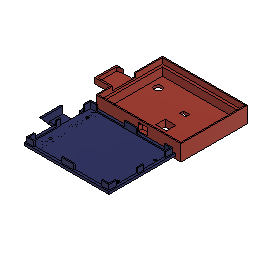
karpiu obudowa (Autodesk Fusion 360 design; units mm, degrees)
part number: Konfiguracja 1
Autodesk Fusion 360 part; units mm, degrees
note: some values were not read from the file. Chosen so that the rebuilt part matches the saved one: which bodies a step acts on; a direction; the layout of a text. Set by a fixed rule: which sketch regions a step uses.
sketch "Szkic1" plane through (0, 0, 0) normal (0, 0, 1) x (1, 0, 0)
  line L0 (65, 50) -> (-65, 50)
  line L1 (-65, 50) -> (-65, -50)
  line L2 (-65, -50) -> (65, -50)
  line L3 (65, -50) -> (65, 50)
  line L4 (-69, -54) -> (69, -54)
  line L5 (69, -54) -> (69, 54)
  line L6 (69, 54) -> (-69, 54)
  line L7 (-69, 54) -> (-69, -54)
  line L8 (-65, 28.5) -> (-91.3384, 28.5)
  line L9 (-91.3384, 28.5) -> (-91.3384, -1.5)
  line L10 (-91.3384, -1.5) -> (-65, -1.5)
  line L11 (-69, 31) -> (-95, 31)
  line L12 (-95, 31) -> (-95, -4)
  line L13 (-95, -4) -> (-69, -4)
  dimension "d100" = 35
  dimension "d101" = 30
  dimension "d102" = 2.5
  dimension "d103" = 100
  dimension "d104" = 130
  constraint horizontal L0
  constraint vertical L1
  constraint horizontal L2
  constraint vertical L3
  constraint horizontal L4
  constraint vertical L5
  constraint horizontal L6
  constraint vertical L7
  constraint coincident L1 L8.start
  constraint perpendicular L7 L8
  constraint perpendicular L8 L9
  constraint coincident L1 L10.end
  constraint perpendicular L1 L10
  constraint coincident L7 L11.start
  constraint perpendicular L7 L11
  constraint perpendicular L8 L12
  constraint coincident L7 L13.end
  constraint perpendicular L7 L13
  measures "d100" distance of L11.end L12.end
  measures "d101" distance of L8.end L9.end
  measures "d102" distance of L10 L13
  measures "d103" distance of L0.start L2.end
  measures "d104" distance of L1.end L2.end
extrude "Wyciągnięcie proste1" add sketch "Szkic1" along normal blind 25 contours L0 L1 L2 L3 L4 L5 L6 L7 L8 L10 | L7 L8 L9 L10 L11 L12 L13 makes body 1
sketch "Szkic2" plane through (0, 0, 25) normal (0, 0, 1) x (-1, 0, 0)
  line L0 (65, 1.5) -> (91.3384, 1.5)
  line L1 (91.3384, 1.5) -> (91.3384, -28.5)
  line L2 (91.3384, -28.5) -> (65, -28.5)
  line L3 (65, -28.5) -> (65, -50)
  line L4 (65, -50) -> (-65, -50)
  line L5 (-65, -50) -> (-65, 50)
  line L6 (-65, 50) -> (65, 50)
  line L7 (65, 50) -> (65, 1.5)
  line L8 (95, 4) -> (69, 4)
  line L9 (69, 4) -> (69, 54)
  line L10 (69, 54) -> (-69, 54)
  line L11 (-69, 54) -> (-69, -54)
  line L12 (-69, -54) -> (69, -54)
  line L13 (69, -54) -> (69, -31)
  line L14 (69, -31) -> (95, -31)
  line L15 (95, -31) -> (95, 4)
  line L16 (-17, -26) -> (0, -26)
  line L17 (0, -26) -> (0, -43)
  line L18 (0, -43) -> (-17, -43)
  line L19 (-17, -43) -> (-17, -26)
  constraint horizontal L16
  constraint vertical L17
  constraint horizontal L18
  constraint vertical L19
extrude "Wyciągnięcie proste2" add sketch "Szkic2" against normal blind 3 contours L0 L1 L2 L3 L4 L5 L6 L7 bodies 1
extrude "Wyciągnięcie proste3" add 1 faces at (0, -27.3333, 25) along direction (0, 0, 1) blind 1 on bodies 1 bodies 1
sketch "Szkic3" plane through (0, 0, 0) normal (0, 0, -1) x (1, 0, 0)
  line L0 (-65, 1.5) -> (-65, 50)
  line L1 (-65, 50) -> (65, 50)
  line L2 (65, 50) -> (65, -50)
  line L3 (65, -50) -> (-65, -50)
  line L4 (-65, -50) -> (-65, -28.5)
  line L5 (-91.3384, -28.5) -> (-91.3384, 1.5)
  line L6 (-95, -31) -> (-69, -31)
  line L7 (-69, -31) -> (-69, -54)
  line L8 (-69, -54) -> (69, -54)
  line L9 (69, -54) -> (69, 54)
  line L10 (69, 54) -> (-69, 54)
  line L11 (-69, 54) -> (-69, 4)
sketch "Szkic4" plane through (0, 0, 26) normal (0, 0, 1) x (-1, 0, 0)
  line L0 (0, -43) -> (-17, -43)
  line L1 (-17, -43) -> (-17, -26)
  line L2 (-17, -26) -> (0, -26)
  line L3 (0, -26) -> (0, -43)
  line L4 (95, 4) -> (69, 4)
  line L5 (69, 4) -> (69, 54)
  line L6 (69, 54) -> (-69, 54)
  line L7 (-69, 54) -> (-69, -54)
  line L8 (-69, -54) -> (69, -54)
  line L9 (69, -54) -> (69, -31)
  line L10 (69, -31) -> (95, -31)
  line L11 (95, -31) -> (95, 4)
  line L12 (69, -31) -> (69, 4)
  constraint coincident L9.end L10.start
  constraint coincident L4.end L5.start
extrude "Wyciągnięcie proste4" cut sketch "Szkic4" against normal blind 20 contours L4 L10 L11 L12 bodies 1
sketch "Szkic5" plane through (0, 0, 6) normal (0, 0, 1) x (-1, 0, 0)
  line L0 (91.3384, -28.5) -> (69, -28.5)
  line L1 (69, -28.5) -> (69, -31)
  line L2 (69, -31) -> (95, -31)
  line L3 (95, -31) -> (95, 4)
  line L4 (95, 4) -> (69, 4)
  line L5 (69, 4) -> (69, 1.5)
  line L6 (69, 1.5) -> (91.3384, 1.5)
  line L7 (91.3384, 1.5) -> (91.3384, -28.5)
  line L8 (69, -28.5) -> (69, 1.5)
  constraint coincident L0.end L1.start
  constraint coincident L5.end L6.start
extrude "Wyciągnięcie proste5" add sketch "Szkic5" along normal blind 3 separate body contours L0 L6 L7 L8 makes body 2
extrude "Wyciągnięcie proste6" add 1 faces at (-93.7795, 18.5, 6) along direction (0, 0, 1) blind 3 on bodies 1 bodies 1 2
sketch "Szkic6" plane through (-69, 0, 0) normal (-1, 0, 0) x (0, -1, 0)
  line L0 (4, 9) -> (4, 0)
  line L1 (4, 0) -> (54, 0)
  line L2 (54, 0) -> (54, 26)
  line L3 (54, 26) -> (-54, 26)
  line L4 (-54, 26) -> (-54, 0)
  line L5 (-54, 0) -> (-31, 0)
  line L6 (-31, 0) -> (-31, 9)
  line L7 (-31, 9) -> (-28.5, 9)
  line L8 (-28.5, 9) -> (-28.5, 22)
  line L9 (-28.5, 22) -> (1.5, 22)
  line L10 (1.5, 22) -> (1.5, 9)
  line L11 (1.5, 9) -> (4, 9)
  line L12 (-28.5, 9) -> (1.5, 9)
  constraint coincident L7.end L8.start
  constraint coincident L10.end L11.start
sketch "Szkic7" plane through (0, -4, 0) normal (0, -1, 0) x (1, 0, 0)
  line L0 (-95, 9) -> (-95, 0)
  line L1 (-95, 0) -> (-69, 0)
  line L2 (-69, 0) -> (-69, 9)
  line L3 (-69, 9) -> (-95, 9)
  line L4 (-90, 0) -> (-90, -11)
  line L5 (-90, -11) -> (-67, -11)
  line L6 (-67, -11) -> (-67, 0)
  line L7 (-90, 0) -> (-94, 0)
  line L8 (-94, 0) -> (-94, -15)
  line L9 (-94, -15) -> (-63, -15)
  line L10 (-63, -15) -> (-63, 0)
  line L11 (-63, 0) -> (-67, 0)
  constraint coincident L1 L4.start
  constraint perpendicular L1 L4
  constraint perpendicular L4 L5
  constraint perpendicular L5 L6
  constraint coincident L1 L7.end
  constraint perpendicular L1 L8
  constraint perpendicular L8 L9
  constraint perpendicular L9 L10
  constraint perpendicular L6 L11
extrude "Wyciągnięcie proste8" add sketch "Szkic7" against normal blind 35 contours L1 L4 L5 L6 L7 L8 L9 L10 L11 bodies 1
sketch "Szkic8" plane through (0, -4, 0) normal (0, -1, 0) x (1, 0, 0)
  line L0 (-95, 9) -> (-95, 0)
  line L1 (-95, 0) -> (-94, 0)
  line L2 (-94, 0) -> (-94, -15)
  line L3 (-94, -15) -> (-63, -15)
  line L4 (-63, -15) -> (-63, 0)
  line L5 (-63, 0) -> (-65, 0)
  line L6 (-65, 0) -> (-67, 0)
  line L7 (-67, 0) -> (-67, -11)
  line L8 (-67, -11) -> (-90, -11)
  line L9 (-90, -11) -> (-90, 0)
  line L10 (-90, 0) -> (-69, 0)
  line L11 (-69, 0) -> (-69, 9)
  line L12 (-69, 9) -> (-95, 9)
  line L13 (-63, 0) -> (-67, 0)
  line L14 (-90, 0) -> (-94, 0)
  line L15 (-94, 0) -> (-94, 9)
  constraint coincident L4.end L5.start
  constraint coincident L6.end L7.start
  constraint coincident L9.end L10.start
  constraint coincident L1.end L2.start
  constraint coincident L12 L15.end
  constraint perpendicular L12 L15
extrude "Wyciągnięcie proste9" cut sketch "Szkic8" against normal blind 13 contours L0 L1 L12 L15 | L2 L3 L4 L5 L6 L7 L8 L9 L13 L14 bodies 1
extrude "Wyciągnięcie proste10" cut 1 faces at (-94.3333, 9, 6) along direction (0, 1, 0) blind 23 on bodies 1 bodies 1
sketch "Szkic9" plane through (0, 9, 0) normal (0, -1, 0) x (1, 0, 0)
  line L0 (-91.3384, 0) -> (-94, 0)
  line L1 (-94, 0) -> (-94, -15)
  line L2 (-94, -15) -> (-63, -15)
  line L3 (-63, -15) -> (-63, 0)
  line L4 (-67, 0) -> (-67, -11)
  line L5 (-67, -11) -> (-90, -11)
  line L6 (-90, -11) -> (-90, 0)
  line L7 (-90, 0) -> (-91.3384, 0)
  line L8 (-67, 0) -> (-67, -0.1)
  line L9 (-67, -0.1) -> (-63, -0.1)
  line L10 (-63, 0) -> (-67, 0)
  constraint coincident L4.start L8.start
  constraint coincident L4 L8.end
  constraint coincident L3 L9.end
  constraint perpendicular L3 L9
extrude "Wyciągnięcie proste11" cut sketch "Szkic9" against normal blind 30 contours L3 L4 L8 L9 L10 bodies 1
sketch "Szkic10" plane through (0, 0, 22) normal (0, 0, -1) x (1, 0, 0)
  line L0 (-69, 1.5) -> (-69, -28.5)
  line L1 (-69, -28.5) -> (-65, -28.5)
  line L2 (-65, -28.5) -> (-65, -50)
  line L3 (-65, -50) -> (65, -50)
  line L4 (65, -50) -> (65, 50)
  line L5 (65, 50) -> (-65, 50)
  line L6 (-65, 50) -> (-65, 1.5)
  line L7 (-65, 1.5) -> (-69, 1.5)
  line L8 (17, -43) -> (0, -43)
  line L9 (0, -43) -> (0, -26)
  line L10 (0, -26) -> (17, -26)
  line L11 (17, -26) -> (17, -43)
  line L12 (-65, 1.5) -> (-65, -32)
  constraint coincident L6.end L7.start
  constraint coincident L2 L12.end
extrude "Wyciągnięcie proste12" add sketch "Szkic10" along normal blind 16 contours L0 L1 L7 L12 bodies 1
sketch "Szkic11" plane through (0, 0, 0) normal (0, 0, -1) x (1, 0, 0)
sketch "Szkic12" plane through (0, 0, 0) normal (0, 0, -1) x (1, 0, 0)
sketch "Szkic13" plane through (0, 0, -11) normal (0, 0, 1) x (-1, 0, 0)
  line L0 (90, -9) -> (67, -9)
  line L1 (67, -9) -> (67, -31)
  line L2 (67, -31) -> (90, -31)
  line L3 (90, -31) -> (90, -9)
  line L4 (90, -31) -> (67, -31)
  line L5 (67, -31) -> (67, -28)
  line L6 (67, -28) -> (90, -28)
  line L7 (90, -28) -> (90, -31)
  constraint horizontal L4
  constraint vertical L5
  constraint horizontal L6
  constraint vertical L7
  constraint coincident L1 L5.end
  constraint coincident L2.end L3.start
extrude "Wyciągnięcie proste13" add sketch "Szkic13" along normal blind 11 contours L1 L2 L3 L4 L5 L6 L7 bodies 1
sketch "Szkic14" plane through (-94, 0, 0) normal (-1, 0, 0) x (0, -1, 0)
  line L0 (-9, -15) -> (-9, 0)
  line L1 (-9, 0) -> (4, 0)
  line L2 (4, 0) -> (4, 9)
  line L3 (4, 9) -> (-31, 9)
  line L4 (-31, 9) -> (-31, -15)
  line L5 (-31, -15) -> (-9, -15)
  line L6 (-9, -15) -> (4, 0)
  constraint coincident L0.start L5.end
  constraint coincident L1.end L2.start
extrude "Wyciągnięcie proste14" add sketch "Szkic14" against normal blind 3 contours L0 L1 L6 bodies 1
extrude "Wyciągnięcie proste15" cut 1 faces at (-90, 15.3333, -3.6667) along direction (-1, 0, 0) blind 1 on bodies 1 bodies 1
extrude "Wyciągnięcie proste16" cut 1 faces at (-67, 15.3333, -7.3667) along direction (1, 0, 0) blind 1 on bodies 1 bodies 1
sketch "Szkic15" plane through (-63, 0, 0) normal (1, 0, 0) x (0, 1, 0)
  line L0 (31, -0.1) -> (9, -0.1)
  line L1 (9, -0.1) -> (9, -15)
  line L2 (9, -15) -> (31, -15)
  line L3 (31, -15) -> (31, -0.1)
  line L4 (9, -15) -> (2.043, 0.0231)
  line L5 (9, -0.1) -> (2.1, -0.1)
  constraint coincident L1.end L2.start
  constraint coincident L0.end L1.start
  constraint coincident L4 L5.end
  constraint perpendicular L1 L5
extrude "Wyciągnięcie proste17" add sketch "Szkic15" against normal blind 3 contours L1 L4 L5 bodies 1
sketch "Szkic16" plane through (-94, 0, 0) normal (-1, 0, 0) x (0, -1, 0)
  line L0 (4, 0) -> (4, 9)
  line L1 (4, 9) -> (-31, 9)
  line L2 (-31, 9) -> (-31, -15)
  line L3 (-31, -15) -> (-9, -15)
  line L4 (-9, -15) -> (4, 0)
  line L5 (4, 0) -> (-31, 0)
  line L6 (-31, 0) -> (-31, -0.1)
  line L7 (-31, -0.1) -> (4, -0.1)
  line L8 (4, -0.1) -> (4, 0)
  constraint horizontal L5
  constraint vertical L6
  constraint horizontal L7
  constraint vertical L8
  constraint coincident L2 L6.end
  constraint coincident L0.start L4.end
extrude "Wyciągnięcie proste18" cut sketch "Szkic16" against normal blind 51 contours L2 L4 L5 L6 L7 bodies 1 makes body 3 at (-74.3333, 23.6667, -15)
move_body "Przesuń1" bodies 3 to x (1, 0, 0) y (0, 1, 0) z (0, 0, 1) at (0, 0, -6)
sketch "Szkic17" plane through (0, 0, -6.1) normal (0, 0, 1) x (-1, 0, 0)
  line L0 (66, -28) -> (66, -2.1)
  line L1 (66, -2.1) -> (63, -2.1)
  line L2 (63, -2.1) -> (63, -31)
  line L3 (63, -31) -> (94, -31)
  line L4 (69, -31) -> (69, -54)
  line L5 (69, -54) -> (-69, -54)
  line L6 (-69, -54) -> (-69, 54)
  line L7 (-69, 54) -> (69, 54)
  line L8 (69, 54) -> (69, -2)
  line L9 (69, -2) -> (66, -2.1)
  line L10 (91, -28) -> (66, -28)
  line L11 (94, -31) -> (94, 3.9133)
  line L12 (94, 3.9133) -> (91, 3.9133)
  line L13 (91, 3.9133) -> (91, -28)
  constraint coincident L3 L4.start
  constraint perpendicular L3 L4
  constraint perpendicular L4 L5
  constraint perpendicular L5 L6
  constraint perpendicular L6 L7
  constraint perpendicular L7 L8
  constraint coincident L0.end L1.start
extrude "Wyciągnięcie proste19" add sketch "Szkic17" against normal blind 2 separate body contours L1 L2 L3 L4 L5 L6 L7 L8 L9 makes body 4
extrude "Wyciągnięcie proste20" add 1 faces at (-63, 11.7333, -6.7667) along direction (-1, 0, 0) blind 3 on bodies 4 bodies 3 4
sketch "Szkic18" plane through (0, 0, -6.1) normal (0, 0, 1) x (-1, 0, 0)
  line L0 (66, -2.1) -> (69, -2)
  line L1 (69, -2) -> (69, 54)
  line L2 (69, 54) -> (-69, 54)
  line L3 (-69, 54) -> (-69, -54)
  line L4 (-69, -54) -> (69, -54)
  line L5 (69, -54) -> (69, -31)
  line L6 (66, -28) -> (66, -2.1)
  line L7 (-65, 50) -> (65, 50)
  line L8 (65, 50) -> (65, -50)
  line L9 (65, -50) -> (-65, -50)
  line L10 (-65, -50) -> (-65, 50)
  line L11 (69, -31) -> (69, -28)
  line L12 (69, -28) -> (65, -28)
  line L13 (69, -2) -> (65, -2)
  line L14 (69, -31) -> (94, -31)
  line L15 (94, -31) -> (94, 3.9133)
  line L16 (94, 3.9133) -> (91, 3.9133)
  line L17 (91, 3.9133) -> (91, -28)
  line L18 (91, -28) -> (66, -28)
  constraint horizontal L7
  constraint vertical L8
  constraint horizontal L9
  constraint vertical L10
  constraint coincident L5.end L11.start
  constraint coincident L8 L12.end
  constraint perpendicular L8 L12
  constraint coincident L0.end L1.start
  constraint coincident L8 L13.end
  constraint perpendicular L8 L13
extrude "Wyciągnięcie proste21" add sketch "Szkic18" along normal blind 2 contours L1 L2 L3 L4 L5 L7 L8 L9 L10 L11 L12 L13 L18 bodies 3
sketch "Szkic19" plane through (0, 0, -4.1) normal (0, 0, 1) x (-1, 0, 0)
  line L0 (69, 54) -> (-69, 54)
  line L1 (-69, 54) -> (-69, -54)
  line L2 (-69, -54) -> (69, -54)
  line L3 (69, -54) -> (69, -28)
  line L4 (69, -28) -> (65, -28)
  line L5 (65, -28) -> (65, -50)
  line L6 (65, -50) -> (-65, -50)
  line L7 (-65, -50) -> (-65, 50)
  line L8 (-65, 50) -> (65, 50)
  line L9 (65, 50) -> (65, -2)
  line L10 (65, -2) -> (69, -2)
  line L11 (69, -2) -> (69, 54)
  line L12 (67, -52) -> (-67, -52)
  line L13 (-67, -52) -> (-67, 52)
  line L14 (-67, 52) -> (67, 52)
  line L15 (67, 52) -> (67, -52)
  constraint horizontal L12
  constraint vertical L13
  constraint horizontal L14
  constraint vertical L15
extrude "Wyciągnięcie proste22" add sketch "Szkic19" along normal blind 8 contours L4 L5 L6 L7 L8 L9 L10 L12 L13 L14 L15 bodies 3
sketch "Szkic20" plane through (0, 0, 3.9) normal (0, 0, 1) x (-1, 0, 0)
  line L0 (67, -28) -> (65, -28)
  line L1 (65, -28) -> (65, -50)
  line L2 (65, -50) -> (-65, -50)
  line L3 (-65, -50) -> (-65, 50)
  line L4 (-65, 50) -> (65, 50)
  line L5 (65, 50) -> (65, -2)
  line L6 (65, -2) -> (67, -2)
  line L7 (67, -2) -> (67, 52)
  line L8 (67, 52) -> (-67, 52)
  line L9 (-67, 52) -> (-67, -52)
  line L10 (-67, -52) -> (67, -52)
  line L11 (67, -52) -> (67, -28)
  line L12 (65, 40) -> (67, 40)
  line L13 (55, 50) -> (55, 52)
  line L14 (-55, 50) -> (-55, 52)
  line L15 (-65, 40) -> (-67, 40)
  line L16 (-65, -40) -> (-67, -40)
  line L17 (-55, -50) -> (-55, -52)
  line L18 (55, -50) -> (55, -52)
  line L19 (65, -40) -> (67, -40)
  line L20 (10, -52) -> (10, -50)
  line L21 (-10, -52) -> (-10, -50)
  line L22 (10, 50) -> (10, 52)
  line L23 (-10, 50) -> (-10, 52)
  line L24 (-65, 5) -> (-67, 5)
  line L25 (-65, -5) -> (-67, -5)
  line L26 (65, 5) -> (67, 5)
  constraint coincident L5 L12.start
  constraint coincident L7 L12.end
  constraint perpendicular L7 L12
  constraint coincident L4 L13.start
  constraint coincident L8 L13.end
  constraint perpendicular L8 L13
  constraint coincident L4 L14.start
  constraint coincident L8 L14.end
  constraint perpendicular L8 L14
  constraint coincident L3 L15.start
  constraint coincident L9 L15.end
  constraint perpendicular L9 L15
  constraint coincident L3 L16.start
  constraint coincident L9 L16.end
  constraint perpendicular L9 L16
  constraint coincident L2 L17.start
  constraint coincident L10 L17.end
  constraint perpendicular L10 L17
  constraint coincident L2 L18.start
  constraint coincident L10 L18.end
  constraint perpendicular L10 L18
  constraint coincident L1 L19.start
  constraint midpoint L11 L19.end
  constraint perpendicular L11 L19
  constraint coincident L10 L20.start
  constraint coincident L2 L20.end
  constraint perpendicular L2 L20
  constraint coincident L10 L21.start
  constraint coincident L2 L21.end
  constraint perpendicular L2 L21
  constraint coincident L4 L22.start
  constraint coincident L8 L22.end
  constraint perpendicular L8 L22
  constraint coincident L4 L23.start
  constraint coincident L8 L23.end
  constraint perpendicular L8 L23
  constraint coincident L3 L24.start
  constraint coincident L9 L24.end
  constraint perpendicular L9 L24
  constraint coincident L3 L25.start
  constraint coincident L9 L25.end
  constraint perpendicular L3 L25
  constraint coincident L5 L26.start
  constraint coincident L7 L26.end
  constraint perpendicular L7 L26
extrude "Wyciągnięcie proste23" cut sketch "Szkic20" against normal blind 8 contours L0 L1 L11 L19 | L2 L10 L18 L20 | L2 L10 L17 L21 | L3 L9 L16 L25 | L3 L9 L15 L24 | L4 L8 L14 L23 | L4 L8 L13 L22 | L5 L7 L12 L26 bodies 3
sketch "Szkic21" plane through (0, 0, 0) normal (0, 0, -1) x (1, 0, 0)
  line L0 (-91.3384, 1.5) -> (-65, 1.5)
  line L1 (-65, 1.5) -> (-65, 50)
  line L2 (-65, 50) -> (65, 50)
  line L3 (65, 50) -> (65, -50)
  line L4 (65, -50) -> (-65, -50)
  line L5 (-65, -50) -> (-65, -28.5)
  line L6 (-65, -28.5) -> (-91.3384, -28.5)
  line L7 (-91.3384, -28.5) -> (-91.3384, 1.5)
  line L8 (-69, 4) -> (-94, 4)
  line L9 (-94, 4) -> (-94, -31)
  line L10 (-94, -31) -> (-69, -31)
  line L11 (-69, -31) -> (-69, -54)
  line L12 (-69, -54) -> (69, -54)
  line L13 (69, -54) -> (69, 54)
  line L14 (69, 54) -> (-69, 54)
  line L15 (-69, 54) -> (-69, 4)
  line L16 (67.2, 52.2) -> (-67.2, 52.2)
  line L17 (-67.2, 52.2) -> (-67.2, -52.2)
  line L18 (-67.2, -52.2) -> (67.2, -52.2)
  line L19 (67.2, -52.2) -> (67.2, 52.2)
  constraint horizontal L16
  constraint vertical L17
  constraint horizontal L18
  constraint vertical L19
extrude "Wyciągnięcie proste24" cut sketch "Szkic21" against normal blind 9 contours L0 L1 L2 L3 L4 L5 L6 L16 L17 L18 L19 bodies 1
sketch "Szkic22" plane through (0, 0, 6) normal (0, 0, -1) x (1, 0, 0)
  line L0 (-67.2, -28.5) -> (-65, -28.5)
  line L1 (-65, -28.5) -> (-65, 1.5)
  line L2 (-65, 1.5) -> (-67.2, 1.5)
  line L3 (-67.2, 1.5) -> (-91.3384, 1.5)
  line L4 (-91.3384, 1.5) -> (-91.3384, -28.5)
  line L5 (-91.3384, -28.5) -> (-67.2, -28.5)
  line L6 (-67.2, 1.5) -> (-67.2, -28.5)
  constraint coincident L2.end L3.start
  constraint coincident L0.start L5.end
extrude "Wyciągnięcie proste25" cut sketch "Szkic22" against normal blind 3 contours L0 L1 L2 L6 bodies 1
extrude "Wyciągnięcie proste26" cut 1 faces at (0, 31.6667, 24.6667) along direction (-1, 0, 0) blind 0.2 on bodies 1 bodies 1
extrude "Wyciągnięcie proste27" cut 1 faces at (5.5333, 26, 24.6667) along direction (0, -1, 0) blind 0.2 on bodies 1 bodies 1
extrude "Wyciągnięcie proste28" cut 1 faces at (5.5333, 43, 23.3333) along direction (0, 1, 0) blind 0.2 on bodies 1 bodies 1
extrude "Wyciągnięcie proste29" cut 1 faces at (17, 31.6, 24.6667) along direction (1, 0, 0) blind 0.2 on bodies 1 bodies 1
move_body "Przesuń2" bodies 1 to x (1, 0, 0) y (0, -1, 0) z (0, 0, -1) at (0, 117, 26)
move_body "Przesuń3" bodies 3 to x (1, 0, 0) y (0, 1, 0) z (0, 0, 1) at (0, 0, 21)
sketch "Szkic23" plane through (0, 67, 0) normal (0, 1, 0) x (-1, 0, 0)
  line L0 (65, 17) -> (-65, 17)
  line L1 (-65, 17) -> (-65, 4)
  line L2 (-65, 4) -> (65, 4)
  line L3 (65, 4) -> (65, 17)
  line L4 (-14.0231, 21.4989, -2.2) -> (-14.0231, 5, -2.2)
  line L5 (-14.0231, 5, -2.2) -> (0, 5, -2.2)
  line L6 (67.2, 26, -2.2) -> (-67.2, 26, -2.2)
  line L7 (-67.2, 26, -2.2) -> (-67.2, 17, -2.2)
  line L8 (-67.2, 17, -2.2) -> (67.2, 17, -2.2)
  line L9 (67.2, 17, -2.2) -> (67.2, 26, -2.2)
  line L10 (0, 5, -2.2) -> (0, 21.5, -2.2)
  line L11 (0, 21.5, -2.2) -> (-14.0231, 21.4989, -2.2)
sketch "Szkic23 (curves -2.2 mm off its plane)" plane through (0, 64.8, 0) normal (0, 1, 0) x (-1, 0, 0)
  line L0 (-14.0231, 21.4989) -> (-14.0231, 5)
  line L1 (-14.0231, 5) -> (0, 5)
  line L2 (67.2, 26) -> (-67.2, 26)
  line L3 (-67.2, 26) -> (-67.2, 17)
  line L4 (-67.2, 17) -> (67.2, 17)
  line L5 (67.2, 17) -> (67.2, 26)
  line L6 (0, 5) -> (0, 21.5)
  line L7 (0, 21.5) -> (-14.0231, 21.4989)
extrude "Wyciągnięcie proste30" cut sketch "Szkic23 (curves -2.2 mm off its plane)" along normal blind -5.57 and the other way blind -6.569 contours L0 L4 L6 L7 | L0 L1 L4 L6 bodies 1
extrude "Wyciągnięcie proste31" add 1 faces at (9.3487, 64.3333, 5) along direction (0, 0, 1) blind 4.364 on bodies 1 bodies 1
sketch "Szkic28" plane through (0, 0, 12.9) normal (0, 0, -1) x (1, 0, 0)
  line L0 (-69, 54) -> (-69, -2)
  line L1 (-69, -2) -> (-66, -2.1)
  line L2 (-66, -2.1) -> (-66, -3.0262)
  line L3 (-66, -3.0262) -> (-63, -3.0262)
  line L4 (-63, -3.0262) -> (-63, -31)
  line L5 (-63, -31) -> (-69, -31)
  line L6 (-69, -31) -> (-69, -54)
  line L7 (-69, -54) -> (69, -54)
  line L8 (69, -54) -> (69, 54)
  line L9 (69, 54) -> (-69, 54)
  line L10 (-39.2305, -52.3086) -> (-39.2305, 47.6914) construction
  line L11 (-39.2305, 47.6914) -> (-59.2305, 47.6914) construction
  line L12 (-59.2305, 47.6914) -> (-59.2305, -52.3086) construction
  line L13 (-59.2305, -52.3086) -> (-39.2305, -52.3086) construction
  dimension "d74" = 10
  text T0 "KARPIOINATOR" font "Arial" height 10 align left top in box 100 x 20 at (-39.2305, -52.3086) x (0, 1) y (-1, 0) spacing 1 kerned
extrude "Wyciągnięcie proste35" cut sketch "Szkic28" against normal blind 0.754 text T0 bodies 3
sketch "Szkic30" plane through (0, 0, 0) normal (0, 0, -1) x (1, 0, 0)
  line L0 (-69, -63) -> (-69, -171)
  line L1 (-69, -171) -> (69, -171)
  line L2 (69, -171) -> (69, -63)
sketch "Szkic31" plane through (0, 0, 0) normal (0, 0, -1) x (1, 0, 0)
  line L0 (-69, -63) -> (-69, -171)
  line L1 (-69, -171) -> (69, -171)
  line L2 (69, -171) -> (69, -63)
  line L3 (69, -63) -> (-69, -63)
  line L4 (13.1675, -132.8725) -> (3.3508, -132.8725)
  line L5 (3.3508, -132.8725) -> (3.3508, -126.6901)
  line L6 (3.3508, -126.6901) -> (13.1675, -126.6901)
  line L7 (13.1675, -126.6901) -> (13.1675, -132.8725)
  line L8 (17.2, -100.9869) -> (-0.2, -100.9869)
  line L9 (-0.2, -100.9869) -> (-0.2, -83.5869)
  line L10 (-0.2, -83.5869) -> (17.2, -83.5869)
  line L11 (17.2, -83.5869) -> (17.2, -100.9869)
extrude "Wyciągnięcie proste37" cut sketch "Szkic31" against normal blind 21.769 contours L4 L5 L6 L7 bodies 1
sketch "Szkic32" plane through (0, 0, 0) normal (0, 0, -1) x (1, 0, 0)
  line L0 (-69, -63) -> (-69, -171)
  line L1 (-69, -171) -> (69, -171)
  line L2 (69, -171) -> (69, -63)
  line L3 (69, -63) -> (-69, -63)
  circle A0 centre (-50, -145) radius 6
  circle A1 centre (8.8135, -94.4712) radius 26.9
  line L4 (3.3508, -132.8725) -> (3.3508, -126.6901)
  line L5 (3.3508, -126.6901) -> (13.1675, -126.6901)
  line L6 (13.1675, -126.6901) -> (13.1675, -132.8725)
  line L7 (13.1675, -132.8725) -> (3.3508, -132.8725)
  line L8 (17.2, -99.9782) -> (-0.2, -99.9782)
  line L9 (-0.2, -99.9782) -> (-0.2, -82.5782)
  line L10 (-0.2, -82.5782) -> (17.2, -82.5782)
  line L11 (17.2, -82.5782) -> (17.2, -99.9782)
  dimension "d84" = 12
  dimension "d85" = 53.8
  measures "d84" diameter of A0
  measures "d85" diameter of A1
extrude "Wyciągnięcie proste38" add sketch "Szkic32" along normal blind 7 contours A1 bodies 1
extrude "Wyciągnięcie proste39" cut sketch "Szkic32" against normal blind 41.04 contours A0 bodies 1
sketch "Szkic33" plane through (0, 0, 14.9) normal (0, 0, 1) x (-1, 0, 0)
  line L0 (65, -28) -> (66, -28)
  line L1 (66, -28) -> (66, -2.1)
  line L2 (66, -2.1) -> (69, -2)
  line L3 (69, -2) -> (65, -2)
  line L4 (65, -2) -> (65, 50)
  line L5 (65, 50) -> (-65, 50)
  line L6 (-65, 50) -> (-65, -50)
  line L7 (-65, -50) -> (65, -50)
  line L8 (65, -50) -> (65, -28)
  circle A0 centre (55, -35) radius 2
  circle A1 centre (-60, -30) radius 2
  circle A2 centre (55, 25) radius 2
  circle A3 centre (-60, 30) radius 2
  dimension "d90" = 4
  dimension "d91" = 4
  dimension "d92" = 4
  dimension "d93" = 4
  measures "d90" diameter of A0
  measures "d91" diameter of A1
  measures "d92" diameter of A2
  measures "d93" diameter of A3
extrude "Wyciągnięcie proste40" cut sketch "Szkic33" against normal blind 5.741 contours A0 | A1 | A2 | A3 bodies 3
sketch "Szkic36" plane through (0, 0, 0) normal (0, 0, -1) x (1, 0, 0)
  line L0 (56.3245, -64.5362) -> (56.3245, -170.6292) construction
  line L1 (56.3245, -170.6292) -> (66.9858, -170.6292) construction
  line L2 (66.9858, -170.6292) -> (66.9858, -64.5362) construction
  line L3 (66.9858, -64.5362) -> (56.3245, -64.5362) construction
  dimension "d96" = 9
  text T0 "KARPIOINATOR" font "Arial" height 9 bold align centre bottom in box 106.0931 x 10.6613 at (56.3245, -64.5362) x (0, -1) y (1, 0) spacing 1 kerned
extrude "Wyciągnięcie proste41" cut sketch "Szkic36" against normal blind 2.398 text T0 bodies 1
extrude "Wyciągnięcie proste42" cut 1 faces at (-75.3333, 28, 7.6333) along direction (0, 1, 0) blind 7.405 on bodies 3 bodies 3
extrude "Wyciągnięcie proste43" cut 1 faces at (11.4, 79.6521, 0) along direction (0, 0, -1) blind 151.178 on bodies 1 bodies 1
sketch "Szkic37" plane through (0, 0, 20) normal (0, 0, 1) x (-1, 0, 0)
  line L0 (67.2, -88.5) -> (67.2, -118.5)
  line L1 (67.2, -118.5) -> (91.3384, -118.5)
  line L2 (91.3384, -118.5) -> (91.3384, -88.5)
  line L3 (91.3384, -88.5) -> (67.2, -88.5)
  line L4 (91, -118.5) -> (67.2, -118.5)
  line L5 (67.2, -125.4479) -> (67.2, -118.5)
  line L6 (67.2, -125.4479) -> (91, -118.5)
  constraint coincident L0.end L1.start
  constraint perpendicular L0 L4
  constraint perpendicular L1 L5
extrude "Wyciągnięcie proste44" cut sketch "Szkic37" along normal blind 22.349 contours L1 L4 L5 L6 bodies 1
extrude "Wyciągnięcie proste45" add 1 faces at (-43.3333, 67, 10.1213) along direction (0, 1, 0) blind 2 on bodies 1 bodies 1
extrude "Wyciągnięcie proste46" add 1 faces at (-21.6667, 167, 12.6667) along direction (0, -1, 0) blind 2 on bodies 1 bodies 1
extrude "Wyciągnięcie proste47" add 1 faces at (-65, 133, 12.6667) along direction (1, 0, 0) blind 2 on bodies 1 bodies 1
extrude "Wyciągnięcie proste48" add 1 faces at (65, 133, 8.3333) along direction (-1, 0, 0) blind 2 on bodies 1 bodies 1
extrude "Wyciągnięcie proste49" add 1 faces at (5.6, 73.8, 0.3333) along direction (0, 1, 0) blind 17.387 on bodies 1 bodies 1
extrude "Wyciągnięcie proste50" cut 1 faces at (5.6, 97.0521, 0) along direction (0, 0, 1) blind 551.263 on bodies 1 bodies 1
move_face "Odsuń powierzchnie1" offset -6.606 1 faces at (11.4, 99.9782, -3.3333) on bodies 1
equation "d75 = 'KARPIOINATOR'"
equation "d97 = 'KARPIOINATOR'"
named bodies: "dolna"
